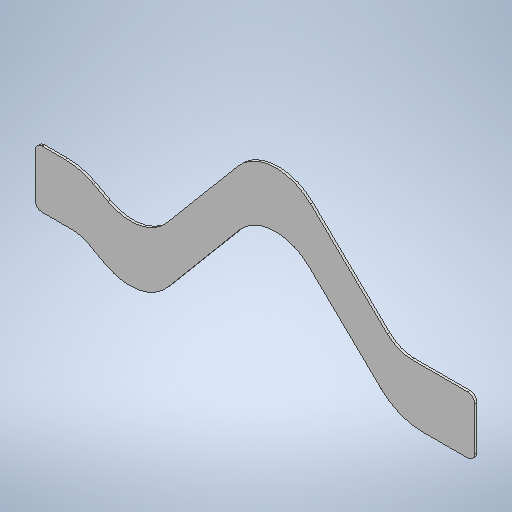
# Autodesk Inventor part: Offset
Saved by Autodesk Inventor 2025 (Build 290162000, 162)
## iProperties
Created: 2024-07-11
Part Number: Offset
Material: Generic
Document SubType Name: Modeling
Designer: usaid
Density: 1 g/cm^3
Appearance: Default
Author: usaid
Autodesk Inventor part; units mm, degrees
ref_plane "YZ Plane" through (0, 0, 0) normal (1, 0, 0) x (0, 1, 0)
ref_plane "XZ Plane" through (0, 0, 0) normal (0, 1, 0) x (-1, 0, 0)
ref_plane "XY Plane" through (0, 0, 0) normal (0, 0, 1) x (1, 0, 0)
sketch "Sketch1" plane through (0, 0, 0) normal (0, 0, 1) x (1, 0, 0)
  arc A0 (0, 3) -> (3, 0) centre (3.0011, 3.0011) ccw
  line L0 (3, 0) -> (15.44, 0)
  arc A1 (22.577, -1.806) -> (15.44, 0) centre (15.444, -14.9894) ccw
  line L1 (22.577, -1.806) -> (29.869, -5.751)
  arc A2 (29.869, -5.751) -> (55.947, -0.778) centre (39.8598, 12.7202) ccw
  line L2 (55.947, -0.778) -> (85.929, 34.955)
  arc A3 (115.145, 36.485) -> (85.929, 34.955) centre (101.2502, 22.1018) ccw
  line L3 (115.145, 36.485) -> (145.651, 7.018)
  arc A4 (145.651, 7.018) -> (163.02, 0) centre (163.0155, 24.9912) ccw
  line L4 (163.02, 0) -> (182, 0)
  arc A5 (182, 0) -> (185, 3) centre (181.9989, 3.0011) ccw
  line L5 (0, 3) -> (0, 21.1)
  arc A6 (3, 24.1) -> (0, 21.1) centre (3.0011, 21.0989) ccw
  line L6 (3, 24.1) -> (12.73, 24.1)
  arc A7 (24.609, 21.097) -> (12.73, 24.1) centre (12.7244, -0.9184) ccw
  line L7 (24.609, 21.097) -> (30.766, 17.772)
  arc A8 (30.766, 17.772) -> (55.59, 22.514) centre (40.2694, 35.3692) ccw
  line L8 (55.59, 22.514) -> (85.294, 57.909)
  arc A9 (115.968, 59.516) -> (85.294, 57.909) centre (101.3803, 44.4098) ccw
  line L9 (115.968, 59.516) -> (148.28, 28.31)
  arc A10 (148.28, 28.31) -> (158.7, 24.1) centre (158.6991, 39.0977) ccw
  line L10 (158.7, 24.1) -> (182, 24.1)
  arc A11 (185, 21.1) -> (182, 24.1) centre (181.9989, 21.0989) ccw
  line L11 (185, 21.1) -> (185, 3)
  constraints: 24 end point, 24 point on circle, 12 centre point
extrude "Extrusion1" add sketch "Sketch1" along normal mid plane 1
body "Solid1"
